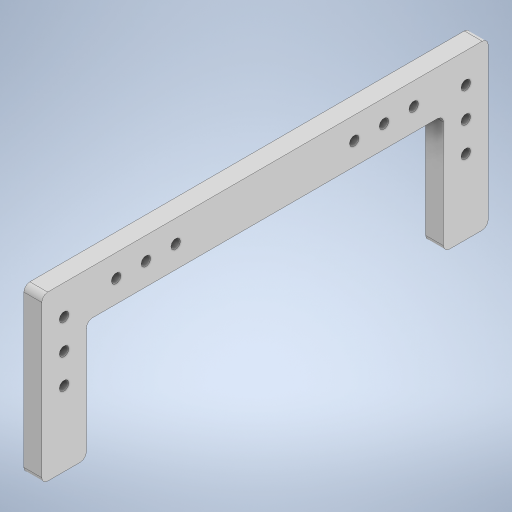
# Autodesk Inventor part: 射出_受け身
Saved by Autodesk Inventor 2023 (Build 270158000, 158)
## iProperties
Created: 2022-04-20
Part Number: 射出_受け身
Material: 一般
Document SubType Name: Modeling
Designer: yuta
Density: 1 g/cm^3
Appearance: 既定
Author: yuta
Autodesk Inventor part; units mm, degrees
ref_plane "YZ Plane" through (0, 0, 0) normal (1, 0, 0) x (0, 1, 0)
ref_plane "XZ Plane" through (0, 0, 0) normal (0, 1, 0) x (-1, 0, 0)
ref_plane "XY Plane" through (0, 0, 0) normal (0, 0, 1) x (1, 0, 0)
sketch "スケッチ1" plane through (0, 0, 0) normal (1, 0, 0) x (0, 1, 0)
  line L0 (0, 0) -> (15, 0)
  line L1 (15, 0) -> (15, -150)
  line L2 (15, -150) -> (0, -150)
  line L3 (0, -150) -> (0, 0)
  line L4 (0, 0) -> (-40, 0)
  line L5 (-40, 0) -> (-40, -15)
  line L6 (-40, -15) -> (0, -15)
  line L7 (0, -15) -> (0, 0)
  line L8 (0, -150) -> (-40, -150)
  line L9 (-40, -150) -> (-40, -135)
  line L10 (-40, -135) -> (0, -135)
  line L11 (0, -135) -> (0, -150)
  dimension "d0" = 15
  dimension "d1" = 150
  dimension "d2" = 40
  dimension "d3" = 15
  dimension "d4" = 40
  dimension "d5" = 15
  constraints: 24 end point, 6 parallel, 3 horizontal, 3 perpendicular
  measures "d0" distance of L1.end L2.end
  measures "d1" distance of L0.end L1.end
  measures "d2" distance of L6.end L5.end
  measures "d3" distance of L5.end L4.end
  measures "d4" distance of L9.end L10.end
  measures "d5" distance of L8.end L9.end
extrude "押し出し1" add sketch "スケッチ1" along normal blind 6
sketch "スケッチ2" plane through (6, 0, 0) normal (1, 0, 0) x (0, 0, -1)
  line L0 (150, 15) -> (0, 15) projected
  line L1 (0, 15) -> (0, -40) projected
  line L2 (75, 15) -> (75, -40) construction
  point P0 (0, 0)
  point P1 (7.5, 5)
  point P2 (7.5, -5)
  point P3 (7.5, -15)
  point P4 (25, 7.5)
  point P5 (35, 7.5)
  point P6 (45, 7.5)
  point P7 (142.5, 5)
  point P8 (142.5, -5)
  point P9 (142.5, -15)
  point P10 (125, 7.5)
  point P11 (115, 7.5)
  point P12 (105, 7.5)
  dimension "d8" = 10
  dimension "d9" = 7.5
  dimension "d10" = 10
  dimension "d11" = 10
  dimension "d12" = 7.5
  dimension "d13" = 25
  dimension "d14" = 10
  dimension "d15" = 10
  constraints: 6 symmetric about line, 2 end point, 1 midpoint, 1 vertical
  measures "d8" distance from line of L0 point (7.5, 5)
  measures "d9" distance from line of L1 point (7.5, 5)
  measures "d10" distance of point (7.5, 5) point (7.5, -5)
  measures "d11" distance of point (7.5, -5) point (7.5, -15)
  measures "d12" distance from line of L0 point (25, 7.5)
  measures "d13" distance from line of L1 point (25, 7.5)
  measures "d14" distance of point (25, 7.5) point (35, 7.5)
  measures "d15" distance of point (35, 7.5) point (45, 7.5)
hole "穴1" at (6, 5, -7.5) at (6, -5, -7.5) at (6, -15, -7.5) at (6, 7.5, -25) at (6, 7.5, -35) at (6, 7.5, -45) at (6, -15, -142.5) at (6, -5, -142.5) at (6, 5, -142.5) at (6, 7.5, -125) at (6, 7.5, -115) at (6, 7.5, -105) direction (-1, 0, 0) diameter 3.2 end through all
fillet "フィレット1" radius 2 8 edges at (3, 15, 0) (3, -40, -135) (3, 15, -150) (3, -40, -150) (3, 0, -15) (3, -40, -15) (3, -40, 0) (3, 0, -135)
